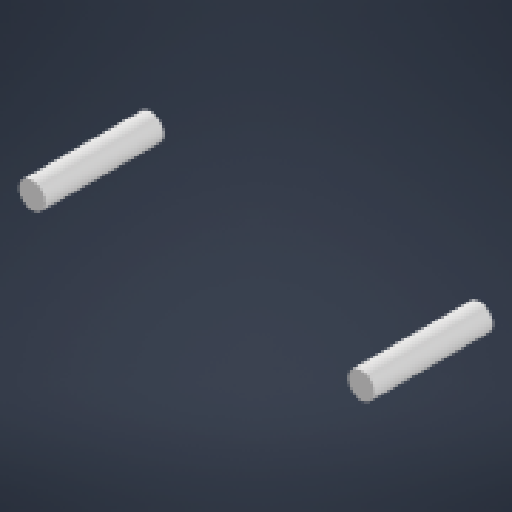
# Autodesk Inventor part: Pieza17
Saved by Autodesk Inventor 2024 (Build 280153000, 153)
## iProperties
Created: 2023-05-13
Part Number: Pieza17
Material: Genérico
Document SubType Name: Modeling
Designer: javie
Density: 1 g/cm^3
Appearance: Valor por defecto
Author: javie
Autodesk Inventor part; units mm, degrees
ref_plane "YZ Plane" through (0, 0, 0) normal (1, 0, 0) x (0, 1, 0)
ref_plane "XZ Plane" through (0, 0, 0) normal (0, 1, 0) x (-1, 0, 0)
ref_plane "XY Plane" through (0, 0, 0) normal (0, 0, 1) x (1, 0, 0)
sketch "Boceto1" plane through (0, 0, 0) normal (0, 0, 1) x (1, 0, 0)
  circle A0 centre (-124.4, 7.2371) radius 2
  circle A1 centre (-174.2, 7.2371) radius 2
  point P0 (0, 0)
  dimension "d0" = 4
  dimension "d2" = 124.4
  dimension "d3" = 174.2
  constraints: 2 centre point
  measures "d0" diameter of A0
  measures "d2" horizontal distance of A0.centre point (0, 0)
  measures "d3" horizontal distance of A1.centre point (0, 0)
extrude "Extrusión1" add sketch "Boceto1" along normal blind 18
